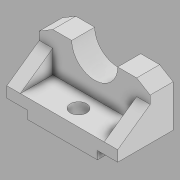
# Autodesk Inventor part: Pieza1
Saved by Autodesk Inventor 2020 (Build 240168000, 168)
## iProperties
Created: 2019-08-16
Part Number: Pieza1
Material: Genérico
Document SubType Name: Modeling
Designer: gerar
Density: 1 g/cm^3
Appearance: Valor por defecto
Author: gerar
Autodesk Inventor part; units mm, degrees
ref_plane "YZ Plane" through (0, 0, 0) normal (1, 0, 0) x (0, 1, 0)
ref_plane "XZ Plane" through (0, 0, 0) normal (0, 1, 0) x (-1, 0, 0)
ref_plane "XY Plane" through (0, 0, 0) normal (0, 0, 1) x (1, 0, 0)
sketch "Boceto1" plane through (0, 0, 0) normal (0, 0, 1) x (1, 0, 0)
  line L0 (0, 0) -> (164, 0)
  line L1 (164, 0) -> (164, 86)
  line L2 (164, 86) -> (0, 86)
  line L3 (0, 86) -> (0, 0)
  dimension "d0" = 164
  dimension "d1" = 86
  constraints: 8 end point, 2 parallel, 1 horizontal, 1 perpendicular
  measures "d0" distance of L2.end L1.end
  measures "d1" distance of L1.end L0.end
extrude "Base" add sketch "Boceto1" along normal blind 82
sketch "Boceto2" plane through (0, 0, 82) normal (0, 0, 1) x (1, 0, 0)
  line L0 (0, 0) -> (164, 0) projected
  line L1 (164, 0) -> (134, 0)
  line L2 (134, 0) -> (134, 12)
  line L3 (134, 12) -> (164, 12)
  line L4 (164, 12) -> (164, 0)
  dimension "d4" = 30
  dimension "d5" = 12
  constraints: 8 end point, 2 parallel, 1 horizontal, 1 perpendicular
  measures "d4" distance of L2.end L3.end
  measures "d5" distance of L1.end L2.end
extrude "Orificio_Inferior_Derecho" cut sketch "Boceto2" against normal blind 82
sketch "Boceto3" plane through (0, 0, 82) normal (0, 0, 1) x (1, 0, 0)
  line L0 (0, 86) -> (0, 0) projected
  line L1 (0, 0) -> (30, 0)
  line L2 (30, 0) -> (30, 12)
  line L3 (30, 12) -> (0, 12)
  line L4 (0, 12) -> (0, 0)
  dimension "d8" = 30
  dimension "d9" = 12
  constraints: 8 end point, 2 parallel, 1 horizontal, 1 perpendicular
  measures "d8" distance of L3.end L2.end
  measures "d9" distance of L2.end L1.end
extrude "Orificio_Inferior_Izquierdo" cut sketch "Boceto3" against normal blind 82
sketch "Boceto5" plane through (0, 0, 0) normal (0, 0, -1) x (-1, 0, 0)
  line L0 (-164, 86) -> (0, 86) projected
  arc A0 (-116, 86) -> (-48, 86) centre (-82, 86) ccw
  point P0 (0, 0)
  dimension "d15" = 68
  constraints: 2 point on circle, 2 point on line, 1 centre point, 1 midpoint
  measures "d15" diameter of A0
extrude "Medio_Círculo" cut sketch "Boceto5" against normal blind 34
sketch "Boceto7" plane through (0, 0, 82) normal (0, 0, 1) x (1, 0, 0)
  line L0 (0, 118.5619) -> (0, 23.764) construction
  line L1 (164, 118.5619) -> (164, 23.764) construction
  line L2 (164, 12) -> (164, 86) projected
  line L3 (0, 86) -> (0, 12) projected
  line L4 (202.848, 28) -> (-57.2499, 28) construction
  line L5 (30, 0) -> (134, 0) projected
  line L6 (164, 86) -> (0, 86) projected
  line L7 (0, 86) -> (164, 86)
  line L8 (164, 86) -> (164, 28)
  line L9 (164, 28) -> (0, 28)
  line L10 (0, 28) -> (0, 86)
  point P0 (0, 0)
  dimension "d23" = 0
  dimension "d24" = 0
  dimension "d25" = 28
  constraints: 14 end point, 4 point on line, 2 horizontal, 2 parallel, 2 vertical, 1 perpendicular
  measures "d23" distance between parallel lines of L2 L1
  measures "d24" distance between parallel lines of L3 L0
  measures "d25" distance between parallel lines of L5 L4
extrude "Hueco" cut sketch "Boceto7" against normal blind 48
sketch "Boceto8" plane through (134, 0, 0) normal (0, -1, 0) x (1, 0, 0)
  line L0 (-150.3038, 58) -> (47.6348, 58) construction
  line L1 (-52, -16.1765) -> (-52, 95.9123) construction
  line L2 (30, 82) -> (30, 0) projected
  line L3 (-104, 82) -> (0, 82) projected
  circle A0 centre (-52, 58) radius 12
  point P0 (-134, 0)
  dimension "d28" = 82
  dimension "d29" = 24
  dimension "d30" = 24
  constraints: 4 end point, 2 point on line, 1 centre point, 1 horizontal, 1 vertical
  measures "d28" distance between parallel lines of L2 L1
  measures "d29" distance between parallel lines of L3 L0
  measures "d30" diameter of A0
extrude "Círculo" cut sketch "Boceto8" against normal blind 28
sketch "Boceto9" plane through (164, 12, 0) normal (1, 0, 0) x (0, 0, -1)
  line L0 (-92.1417, 50) -> (23.5619, 50) construction
  line L1 (-34, 16) -> (-82, 16) projected
  line L2 (-34, 74) -> (-34, 16) projected
  line L3 (-34, 50) -> (-82, 16)
  line L4 (-34, 16) -> (-34, 50)
  line L5 (-34, 16) -> (-82, 16)
  point P0 (0, -12)
  dimension "d33" = 34
  constraints: 8 end point, 2 point on line, 1 collinear, 1 horizontal, 1 vertical
  measures "d33" distance between parallel lines of L0 L1
extrude "Triángulo_Derecho" add sketch "Boceto9" against normal blind 20
sketch "Boceto10" plane through (0, 12, 0) normal (-1, 0, 0) x (0, 0, 1)
  line L0 (-15.7199, 50) -> (95.5491, 50) construction
  line L1 (82, 16) -> (34, 16) projected
  line L2 (34, 16) -> (34, 50) projected
  line L3 (34, 50) -> (34, 16)
  line L4 (82, 16) -> (34, 16) projected
  line L5 (34, 16) -> (82, 16)
  line L6 (82, 16) -> (34, 50)
  point P0 (0, -12)
  dimension "d36" = 34
  constraints: 8 end point, 2 collinear, 1 horizontal
  measures "d36" distance between parallel lines of L0 L1
extrude "Triángulo_Izquierdo" add sketch "Boceto10" against normal blind 20
sketch "Boceto11" plane through (0, 0, 0) normal (0, 0, -1) x (-1, 0, 0)
  line L0 (-144, 115.7571) -> (-144, -22.8513) construction
  line L1 (-164, 12) -> (-164, 86) projected
  line L2 (-189.9872, 62) -> (67.4285, 62) construction
  line L3 (-30, 0) -> (-134, 0) projected
  line L4 (-116, 86) -> (-164, 86) projected
  line L5 (-189.9872, 86) -> (-164, 86) construction
  line L6 (-197.4576, 74) -> (12.6853, 74) construction
  line L7 (-144, 86) -> (-164, 86)
  line L8 (-164, 86) -> (-164, 62) projected
  line L9 (-164, 86) -> (-164, 74)
  line L10 (-164, 74) -> (-144, 86)
  point P0 (0, 0)
  dimension "d39" = 20
  dimension "d40" = 62
  dimension "d41" = 24
  dimension "d42" = 12
  constraints: 14 end point, 2 collinear, 2 horizontal, 2 point on line, 1 midpoint, 1 vertical
  measures "d39" distance between parallel lines of L1 L0
  measures "d40" distance between parallel lines of L2 L3
  measures "d41" distance between parallel lines of L2 L5
  measures "d42" distance between parallel lines of L6 L5
extrude "Recorte_Superior_Derecho" cut sketch "Boceto11" against normal blind 34
sketch "Boceto12" plane through (0, 0, 0) normal (0, 0, -1) x (-1, 0, 0)
  line L0 (-163.8025, 74) -> (21.144, 74) construction
  line L1 (-20, 114.5089) -> (-20, -16.4312) construction
  line L2 (-48, 86) -> (0, 86) projected
  line L3 (0, 86) -> (0, 12) projected
  line L4 (0, 86) -> (-20, 86)
  line L5 (0, 62) -> (0, 86) projected
  line L6 (0, 74) -> (0, 86)
  line L7 (0, 86) -> (0, 74)
  line L8 (0, 74) -> (-20, 86)
  point P0 (0, 0)
  dimension "d45" = 12
  dimension "d46" = 20
  constraints: 12 end point, 2 point on line, 1 collinear, 1 horizontal, 1 midpoint, 1 perpendicular, 1 vertical
  measures "d45" distance between parallel lines of L0 L2
  measures "d46" distance between parallel lines of L3 L1
extrude "Recorte_Superior_Izquierdo" cut sketch "Boceto12" against normal blind 34
